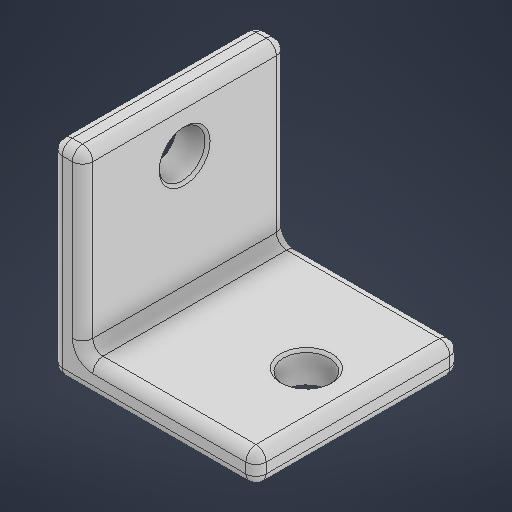
# Autodesk Inventor part: Aquerre
Saved by Autodesk Inventor 2026.2 (Build 302298010, 298A)
## iProperties
Created: 2026-05-02
Part Number: Aquerre
Material: Générique
Document SubType Name: Modeling
Designer: romai
Density: 1 g/cm^3
Appearance: Par défaut
Author: romai
Autodesk Inventor part; units mm, degrees
ref_plane "YZ Plane" through (0, 0, 0) normal (1, 0, 0) x (0, 1, 0)
ref_plane "XZ Plane" through (0, 0, 0) normal (0, 1, 0) x (-1, 0, 0)
ref_plane "XY Plane" through (0, 0, 0) normal (0, 0, 1) x (1, 0, 0)
sketch "Esquisse1" plane through (0, 0, 0) normal (0, 1, 0) x (-1, 0, 0)
  line L0 (-10, 10) -> (10, 10)
  line L1 (10, 10) -> (10, -10)
  line L2 (10, -10) -> (-10, -10)
  line L3 (-10, -10) -> (-10, 10)
  line L4 (-10, 10) -> (10, -10) construction
  line L5 (10, 10) -> (-10, -10) construction
  point P0 (0, 0)
  dimension "d0" = 20
  dimension "d1" = 20
  constraints: 12 end point, 2 midpoint, 2 parallel, 1 horizontal, 1 perpendicular
  measures "d0" distance of L1.end L2.end
  measures "d1" distance of L0.end L1.end
extrude "Extrusion1" add sketch "Esquisse1" along normal blind 3
sketch "Esquisse2" plane through (-10, 0, -10) normal (-1, 0, 0) x (0, 0, 1)
  line L0 (0, 20) -> (20, 20)
  line L1 (20, 20) -> (20, 3)
  line L2 (20, 3) -> (0, 3)
  line L3 (0, 3) -> (0, 20)
  line L4 (0, 20) -> (20, 3) construction
  line L5 (20, 20) -> (0, 3) construction
  line L6 (0, 0) -> (20, 0) projected
  point P0 (10, 0)
  point P1 (10, 11.5)
  dimension "d4" = 20
  dimension "d5" = 17
  dimension "d6" = 3
  constraints: 12 end point, 2 midpoint, 2 parallel, 1 horizontal, 1 perpendicular
  measures "d4" distance of L1.end L2.end
  measures "d5" distance of L0.end L1.end
  measures "d6" distance between parallel lines of L6 L2
extrude "Extrusion2" add sketch "Esquisse2" against normal blind 3
fillet "Congé1" radius 1 18 edges at (10, 3, 0) (1.5, 3, 10) (10, 1.5, 10) (-7, 11.5, 10) (0, 0, 10) (-10, 10, 10) (-10, 0, 0) (-10, 10, -10) (0, 0, -10) (1.5, 3, -10) (-7, 11.5, -10) (10, 1.5, -10) (10, 0, 0) (-7, 3, 0) (-7, 20, 0) (-10, 20, 0) (-8.5, 20, 10) (-8.5, 20, -10)
sketch "Esquisse3" plane through (0, 3, 0) normal (0, 1, 0) x (1, 0, 0)
  line L0 (10, -9) -> (10, 9) projected
  point P0 (0, 0)
  point P1 (5, -0.0654)
  dimension "d24" = 5
  measures "d24" distance from line of point (5, -0.065) L0
hole "Perçage1" at (5, 3, 0.0654) direction (0, -1, 0) diameter 4.5 depth 16.2 tip angle 118 countersink diameter 5 countersink angle 90 clearance for "Vis à tête plate fraisée ISO 2009/7046" size "M4" standard "ISO"
sketch "Esquisse4" plane through (-7, 0, -10) normal (1, 0, 0) x (0, 0, -1)
  line L0 (-1, 20) -> (-19, 20) projected
  line L1 (-20, 19) -> (-20, 4) projected
  point P0 (-10, 0)
  point P1 (-10, 15)
  dimension "d25" = 5
  dimension "d26" = 10
  measures "d25" distance from line of L0 point (-10, 15)
  measures "d26" distance from line of L1 point (-10, 15)
hole "Perçage2" at (-7, 15, 0) direction (-1, 0, 0) diameter 4.5 depth 16.2 tip angle 118 countersink diameter 5 countersink angle 90 clearance for "Vis à tête plate fraisée ISO 2009/7046" size "M4" standard "ISO"
